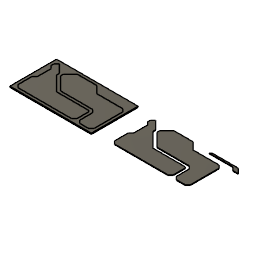
power_supply_side_piece_cyberpunk (Autodesk Fusion 360 design; units mm, degrees)
Autodesk Fusion 360 part; units mm, degrees
sketch "Schizzo1" plane through (0, 0, 0) normal (0, 0, 1) x (1, 0, 0)
  line L0 (0, 0) -> (148, 0)
  line L1 (148, 0) -> (148, 85)
  line L2 (148, 85) -> (0, 85)
  line L3 (0, 85) -> (0, 0)
  line L4 (143, 10) -> (143, 62.0711)
  line L5 (77.9288, 80) -> (42.9288, 80)
  line L6 (5, 75) -> (10, 80)
  line L7 (5, 75) -> (5, 70)
  line L8 (5, 70) -> (10, 65)
  line L9 (10, 65) -> (10, 40)
  line L10 (10, 40) -> (5, 35)
  line L11 (5, 75) -> (5, 70)
  line L12 (5, 35) -> (5, 10)
  line L13 (10, 80) -> (25, 65)
  line L14 (25, 65) -> (25, 60)
  line L15 (25, 60) -> (50.0003, 35)
  line L16 (30, 62.0711) -> (53.5358, 38.5356)
  line L17 (30, 62.0711) -> (30, 67.0711)
  line L18 (30, 67.0711) -> (42.9288, 80)
  line L19 (42.9288, 80) -> (77.9288, 80)
  line L20 (77.9288, 80) -> (90.8578, 67.0711)
  line L21 (138, 67.0711) -> (143, 62.0711)
  line L22 (138, 67.0711) -> (90.8578, 67.0711)
  line L23 (10, 5) -> (5, 10)
  line L24 (138, 5) -> (143, 10)
  line L25 (116.9645, 10) -> (121.9645, 5)
  line L26 (116.9645, 10) -> (116.9645, 33.5356)
  line L27 (111.9645, 38.5356) -> (53.5358, 38.5356)
  line L28 (111.9645, 38.5356) -> (116.9645, 33.5356)
  line L29 (111.9645, 10) -> (111.9645, 31.4645)
  line L30 (109.8934, 33.5356) -> (111.9645, 31.4645)
  line L31 (109.8934, 33.5356) -> (53.5358, 33.5356)
  line L32 (111.9645, 10) -> (106.9645, 5)
  line L33 (10, 5) -> (106.9645, 5)
  line L34 (121.9645, 5) -> (138, 5)
  line L35 (50.0003, 35) -> (51.4647, 33.5356)
  line L36 (51.4647, 33.5356) -> (53.5358, 33.5356)
  line L37 (113.2071, 41.5356) -> (119.0858, 35.6569)
  line L38 (113.2071, 41.5356) -> (69.8324, 41.5356)
  line L39 (119.0858, 35.6569) -> (129.0858, 35.6569)
  line L40 (123.2071, 41.5356) -> (129.0858, 35.6569)
  line L41 (113.2071, 44.5356) -> (72.8324, 44.5356)
  line L42 (123.2071, 41.5356) -> (120.2071, 44.5356)
  line L43 (120.2071, 44.5356) -> (113.2071, 44.5356)
  line L44 (72.8324, 44.5356) -> (69.8324, 41.5356)
  dimension "d1" = 148
  dimension "d2" = 85
  dimension "d4" = 5
  dimension "d5" = 135
  dimension "d6" = -5
  dimension "d7" = 5
  dimension "d8" = 35
  dimension "d11" = 52.0711
  dimension "d12" = 26.0355
  dimension "d16" = -5
  dimension "d19" = 10
  constraint horizontal L0
  constraint vertical L1
  constraint horizontal L2
  constraint vertical L3
  constraint coincident L0.start L3.end
  constraint parallel L7 L11
  constraint parallel L7 L9
  constraint perpendicular L8 L10
  constraint collinear L11 L12
  constraint perpendicular L6 L13
  constraint parallel L9 L14
  constraint vertical L17
  constraint perpendicular L16 L18
  constraint parallel L5 L19
  constraint perpendicular L18 L20
  constraint parallel L21 L23
  constraint perpendicular L26 L27
  constraint collinear L33 L34
  constraint parallel L15 L35
  constraint parallel L31 L36
  constraint horizontal L39
  constraint parallel L40 L42
  constraint parallel L41 L43
  measures "d1" distance of L0.start L0.end
  measures "d2" distance of L0.start L2.end
  measures "d4" distance of L6.start L7.end
  measures "d5" angle of L14 L15
  measures "d7" distance of L16.start L17.end
  measures "d8" distance of L5.end L5.start
  measures "d11" distance of L4.end L4.start
  measures "d12" distance of L4.start L25.start
  measures "d19" distance of L37.end L39.end
extrude "Estrusione1" add sketch "Schizzo1" along normal blind 2 contours L0 L1 L2 L3 | L4 L5 L16 L17 L18 L19 L20 L21 L22 L24 L25 L26 L27 L28 L34 | L6 L7 L8 L9 L10 L11 L12 L13 L14 L15 L23 L29 L30 L31 L32 L33 L35 L36 | L37 L38 L39 L40 L41 L42 L43 L44 makes body 1
extrude "Estrusione2" add sketch "Schizzo1" along normal blind 3 separate body contours L4 L5 L16 L17 L18 L19 L20 L21 L22 L24 L25 L26 L27 L28 L34 | L6 L7 L8 L9 L10 L11 L12 L13 L14 L15 L23 L29 L30 L31 L32 L33 L35 L36 | L37 L38 L39 L40 L41 L42 L43 L44 makes body 2 at (85.4527, 48.0474, 0) makes body 3 at (56.1431, 14.5119, 0)
extrude "Estrusione3" add sketch "Schizzo1" along normal blind 4 separate body contours L37 L38 L39 L40 L41 L42 L43 L44 makes body 4
split_face "DividiFaccia1" 1 faces at (49.3333, 56.6667, 2) by bodies 3 2 on bodies 1
extrude "Estrusione4" cut 2 faces at (85.4527, 48.0474, 0) (56.1431, 14.5119, 0) along direction (0, 0, 1) blind 2 on bodies 2 3 bodies 2 3 4
extrude "Estrusione5" cut 1 faces at (122.7929, 38.6164, 2) along direction (0, 0, 1) blind 1 on bodies 4 bodies 4
move_body "Sposta1" bodies 3 to x (1, 0, 0) y (0, 1, 0) z (0, 0, 1) at (175, 0, -2)
move_body "Sposta2" bodies 2 to x (1, 0, 0) y (0, 1, 0) z (0, 0, 1) at (175, 0, -2)
move_body "Sposta3" bodies 4 to x (1, 0, 0) y (0, 1, 0) z (0, 0, 1) at (215, 35, -3)
equation "d12 = ( 52.0710851846 / 2 ) * 1 mm"
